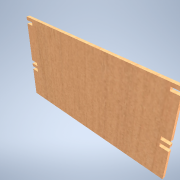
# Autodesk Inventor part: DoosjeVoorkant
Saved by Autodesk Inventor 2021 (Build 250183000, 183)
## iProperties
Created: 2021-03-11
Part Number: DoosjeVoorkant
Material: Wood (Cherry)
Document SubType Name: Modeling
Designer: ZiweZhang
Density: 0.63 g/cm^3
Appearance: Cherry - Natural Low Gloss
Author: ZiweZhang
Autodesk Inventor part; units mm, degrees
ref_plane "YZ Plane" through (0, 0, 0) normal (1, 0, 0) x (0, 1, 0)
ref_plane "XZ Plane" through (0, 0, 0) normal (0, 1, 0) x (-1, 0, 0)
ref_plane "XY Plane" through (0, 0, 0) normal (0, 0, 1) x (1, 0, 0)
sketch "Sketch1" plane through (0, 0, 0) normal (0, 0, 1) x (1, 0, 0)
  line L0 (0, 0) -> (144, 0)
  line L1 (144, 0) -> (144, 77)
  line L2 (144, 77) -> (0, 77)
  line L3 (0, 77) -> (0, 0)
  dimension "d0" = 144
  dimension "d1" = 77
  constraints: 8 end point, 2 parallel, 1 horizontal, 1 perpendicular
  measures "d0" distance of L2.end L1.end
  measures "d1" distance of L1.end L0.end
extrude "Extrusion1" add sketch "Sketch1" along normal blind 3
sketch "Sketch3" plane through (0, 0, 3) normal (0, 0, 1) x (1, 0, 0)
  line L0 (0, 74) -> (7, 74)
  line L1 (7, 74) -> (7, 71)
  line L2 (7, 71) -> (0, 71)
  line L3 (0, 71) -> (0, 74)
  line L4 (137, 74) -> (144, 74)
  line L5 (144, 74) -> (144, 71)
  line L6 (144, 71) -> (137, 71)
  line L7 (137, 71) -> (137, 74)
  line L8 (0, 36) -> (7, 36)
  line L9 (7, 36) -> (7, 33)
  line L10 (7, 33) -> (0, 33)
  line L11 (0, 33) -> (0, 36)
  line L12 (137, 36) -> (144, 36)
  line L13 (144, 36) -> (144, 33)
  line L14 (144, 33) -> (137, 33)
  line L15 (137, 33) -> (137, 36)
  line L16 (7, 30) -> (7, 27)
  line L17 (7, 27) -> (0, 27)
  line L18 (0, 30) -> (7, 30)
  line L19 (0, 27) -> (0, 30)
  line L20 (144, 36) -> (144, 33)
  line L21 (144, 33) -> (137, 33)
  line L22 (137, 36) -> (144, 36)
  line L23 (137, 33) -> (137, 36)
  line L24 (144, 30) -> (144, 27)
  line L25 (144, 27) -> (137, 27)
  line L26 (137, 30) -> (144, 30)
  line L27 (137, 27) -> (137, 30)
  point P0 (0, 0)
  dimension "d27" = 7
  dimension "d28" = 3
  dimension "d31" = 137
  dimension "d34" = 38
  dimension "d41" = 6
  dimension "d44" = 137
  constraints: 56 end point, 4 collinear, 3 horizontal, 3 perpendicular, 2 vertical, 44 other
  measures "d27" distance of L0.start L0.end
  measures "d28" distance of L0.end L1.end
  measures "d31" distance of L0.start L4.start
  measures "d34" distance of L0.start L8.start
  measures "d41" distance of L9.end L16.end
  measures "d44" distance of L9.end L20.end
extrude "Extrusion2" cut sketch "Sketch3" against normal through all
sketch "Sketch4" plane through (0, 0, 3) normal (0, 0, 1) x (1, 0, 0)
  line L0 (47, 70) -> (97, 70)
  line L1 (97, 70) -> (97, 60)
  line L2 (97, 60) -> (47, 60)
  line L3 (47, 60) -> (47, 70)
  line L4 (47, 70) -> (97, 60) construction
  line L5 (97, 70) -> (47, 60) construction
  point P0 (0, 0)
  point P1 (72, 65)
  dimension "d47" = 50
  dimension "d48" = 10
  constraints: 12 end point, 2 midpoint, 2 parallel, 1 horizontal, 1 perpendicular
  measures "d47" distance of L1.end L2.end
  measures "d48" distance of L0.end L1.end
extrude "Extrusion4" cut sketch "Sketch4" against normal blind 1.5
body "Solid1"
